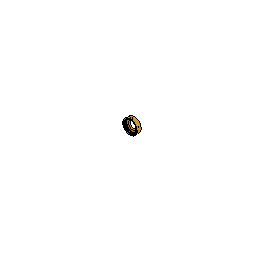
Topper_Interface (Autodesk Fusion 360 design; units mm, degrees)
Autodesk Fusion 360 part; units mm, degrees
sketch "Sketch1" plane through (0, 0, 0) normal (0, 1, 0) x (1, 0, 0)
  circle A0 centre (0, 0) radius 15.5
  circle A1 centre (0, 0) radius 9
  dimension "d62" = 31
  dimension "d63" = 18
  constraint coincident A0.centre A1.centre
  measures "d62" diameter of A0
  measures "d63" diameter of A1
extrude "Extrude1" add sketch "Sketch1" along normal blind 1 from surface at 12
sketch "Sketch2" plane through (0, 12, 0) normal (0, -1, 0) x (1, 0, 0)
  circle A0 centre (0, 0) radius 9
  circle A1 centre (0, 0) radius 15.5
  circle A2 centre (0, 0) radius 13.5
  dimension "d67" = -2
extrude "Extrude2" add sketch "Sketch2" along normal blind 6 contours A1
thread "Thread1" "ISO Metric profile 28.0 M28x2 6H" major diameter 28.2565 minor diameter 26.0224 pitch 2 angle 60 modelled right hand crest width 0.5434 on face at (13.4832, 8, -0.6729) crest through (13.0112, 11.5, 0)
extrude "Extrude3" add 1 faces at (13.2421, 13, -1.2172) along direction (0, 1, 0) blind 2
sketch "Sketch13" plane through (0, 0, 0) normal (0, 0, 1) x (1, 0, 0)
  line L0 (-9, 15) -> (9, 15)
  line L1 (9, 12) -> (-9, 12)
  line L2 (9, 12) -> (7.6706, 15)
  line L3 (9, 15) -> (9, 12)
  dimension "d118" = 66.1
  constraint coincident L1.start L2.start
  constraint coincident L0 L2.end
  constraint coincident L0.end L3.start
  measures "d118" angle of L0 L2
revolve "Revolve2" add sketch "Sketch13" angle 360 about axis through (0, 1.75, 0) along (0, 1, 0)
equation "d118 = 180 deg - 113.9 deg"
named bodies: "Topper_Interface"
